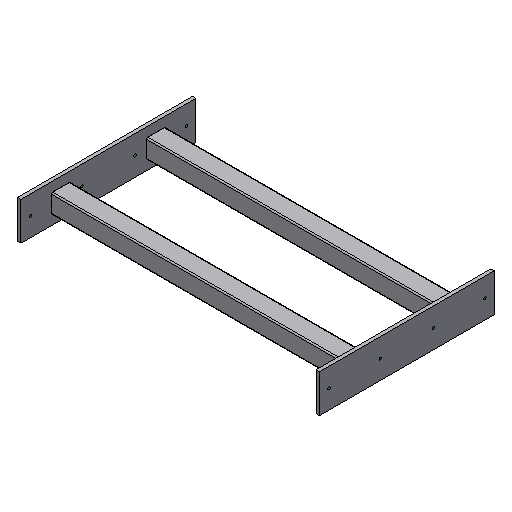
# Autodesk Inventor part: TL20240701-10110CV-031
Saved by Autodesk Inventor 2022.5 (Build 265521000, 521)
## iProperties
Category: DRIVE UNIT ASSY
Company: 현대 트랜시스(대유)
Created: 2023-04-13
Part Number: TL20240701-10110CV-031
Checked By: 김형민
Engr Approved By: 김시현
User Status: 1 x18
Material: SS400
Description: 0
Document SubType Name: Modeling
Mfg Approved By: 호상태
Designer: 정희영
Stock Number: 031
Density: 7.85 g/cm^3
Appearance: Painting-RAL7035
Project: SW PJT
DETAIL: Coveryor Assembly
M/C TITLE: CJ 제일제당 협동로봇 포장시스탬 PILOT 장비
PARTS NAME: Bracket
SPECIFICATION: TA20221101-CV200000-015
DocNumber: 221118_Standard_v1
Folder: .\
VDS_Category: 엔지니어링
Detail Description: Processed products
Title: JOINT
Subject: SW차종 시트조립라인
Author: 정희영
Revision Number: A
Autodesk Inventor part; units mm, degrees
ref_plane "YZ Plane" through (0, 0, 0) normal (1, 0, 0) x (0, 1, 0)
ref_plane "XZ Plane" through (0, 0, 0) normal (0, 1, 0) x (-1, 0, 0)
ref_plane "XY Plane" through (0, 0, 0) normal (0, 0, 1) x (1, 0, 0)
sketch "스케치9" plane through (0, 0, 0) normal (1, 0, 0) x (0, 1, 0)
  line L0 (-50, 230) -> (50, 230)
  line L1 (50, 230) -> (50, -230)
  line L2 (50, -230) -> (-50, -230)
  line L3 (-50, -230) -> (-50, 230)
  line L4 (-50, 230) -> (50, -230) construction
  line L5 (50, 230) -> (-50, -230) construction
  point P0 (0, 0)
  dimension "d40" = 460
  dimension "d41" = 100
  constraints: 12 end point, 2 midpoint, 2 parallel, 1 horizontal, 1 perpendicular
  measures "d40" distance of L0.end L1.end
  measures "d41" distance of L1.end L2.end
extrude "돌출4" add sketch "스케치9" along normal mid plane 9
sketch "스케치10" plane through (4.5, 0, 0) normal (1, 0, 0) x (0, 0, -1)
  line L0 (-150, 25) -> (-100, 25)
  line L1 (-100, 25) -> (-100, -25)
  line L2 (-100, -25) -> (-150, -25)
  line L3 (-150, -25) -> (-150, 25)
  line L4 (100, 25) -> (150, 25)
  line L5 (150, 25) -> (150, -25)
  line L6 (150, -25) -> (100, -25)
  line L7 (100, -25) -> (100, 25)
  line L8 (-101.6, 23.4) -> (-148.4, 23.4)
  line L9 (-148.4, 23.4) -> (-148.4, -23.4)
  line L10 (-148.4, -23.4) -> (-101.6, -23.4)
  line L11 (-101.6, -23.4) -> (-101.6, 23.4)
  line L12 (148.4, 23.4) -> (101.6, 23.4)
  line L13 (101.6, 23.4) -> (101.6, -23.4)
  line L14 (101.6, -23.4) -> (148.4, -23.4)
  line L15 (148.4, -23.4) -> (148.4, 23.4)
  line L16 (230, 50) -> (-230, 50) projected
  point P0 (0, 0)
  dimension "d44" = 50
  dimension "d45" = 50
  dimension "d46" = 1.6
  dimension "d47" = 1.6
  dimension "d48" = 100
  dimension "d49" = 200
  dimension "d50" = 25
  constraints: 32 end point, 8 parallel, 4 perpendicular, 2 equal length, 2 horizontal, 1 collinear, 6 other
  measures "d44" distance of L0.start L0.end
  measures "d45" distance of L2.end L0.start
  measures "d46" distance between parallel lines of L0 L8
  measures "d47" distance between parallel lines of L4 L12
  measures "d48" distance from line of point (0, 0) L1
  measures "d49" distance between parallel lines of L7 L1
  measures "d50" distance between parallel lines of L0 L16
extrude "돌출5" add sketch "스케치10" along normal blind 776 separate body
fillet "모깎기2" radius 1.6 8 edges at (392.5, 23.4, 148.4) (392.5, 23.4, 101.6) (392.5, -23.4, 101.6) (392.5, -23.4, 148.4) (392.5, -23.4, -101.6) (392.5, 23.4, -101.6) (392.5, 23.4, -148.4) (392.5, -23.4, -148.4)
fillet "모깎기3" radius 3.2 8 edges at (392.5, 25, -100) (392.5, 25, -150) (392.5, -25, -100) (392.5, -25, -150) (392.5, -25, 100) (392.5, 25, 100) (392.5, 25, 150) (392.5, -25, 150)
sketch "스케치11" plane through (780.5, 0, 0) normal (1, 0, 0) x (0, 0, -1)
  line L0 (230, 50) -> (-230, 50) projected
  line L1 (230, -50) -> (230, 50) projected
  line L2 (230, 50) -> (-230, 50) projected
  line L3 (-230, 50) -> (-230, -50) projected
  line L4 (-230, -50) -> (230, -50) projected
  point P0 (0, 0)
extrude "돌출6" add sketch "스케치11" along normal blind 9 separate body
sketch "스케치12" plane through (-4.5, 0, 0) normal (-1, 0, 0) x (0, 0, 1)
  line L0 (230, -50) -> (230, 50) projected
  line L1 (-230, 50) -> (-230, -50) projected
  line L2 (-230, -50) -> (230, -50) projected
  point P0 (0, 0)
  point P1 (-205, 0)
  point P2 (-70, 0)
  point P3 (70, 0)
  point P4 (205, 0)
  dimension "d57" = 25
  dimension "d58" = 25
  dimension "d61" = 135
  dimension "d63" = 135
  dimension "d64" = 50
  constraints: 3 horizontal alignment
  measures "d57" distance from line of L0 point (205, 0)
  measures "d58" distance from line of L1 point (-205, 0)
  measures "d61" distance of point (70, 0) point (205, 0)
  measures "d63" distance of point (-70, 0) point (-205, 0)
  measures "d64" distance from line of L2 point (205, 0)
hole "구멍3" at (-4.5, 0, -205) at (-4.5, 0, -70) at (-4.5, 0, 70) at (-4.5, 0, 205) direction (1, 0, 0) diameter 6.647 depth 20 tip angle 118 bodies 1 thread size "M8x1.25" class "6H" standard "ISO Metric profile"
sketch "스케치13" plane through (789.5, 0, 0) normal (1, 0, 0) x (0, 0, -1)
  circle A0 centre (-205, 0) radius 3.3235 projected
  circle A1 centre (-70, 0) radius 3.3235 projected
  circle A2 centre (70, 0) radius 3.3235 projected
  circle A3 centre (205, 0) radius 3.3235 projected
  circle A4 centre (-70, 0) radius 3.3235 projected
  circle A5 centre (70, 0) radius 3.3235 projected
  circle A6 centre (205, 0) radius 3.3235 projected
  point P0 (0, 0)
  point P1 (-70, 0)
  point P2 (70, 0)
  constraints: 4 coincident
hole "구멍4" at (789.5, 0, 205) at (789.5, 0, 70) at (789.5, 0, -70) at (789.5, 0, -205) direction (-1, 0, 0) diameter 6.647 depth 20 tip angle 118 bodies 3 thread size "M8x1.25" class "6H" standard "ISO Metric profile"
equation "\"d42\" = t"
equation "\"d51\" = PLATE_L - 2 * t"
equation "\"d53\" = t"
equation "\"t\" = 9"
equation "\"PLATE_L\" = 794"
